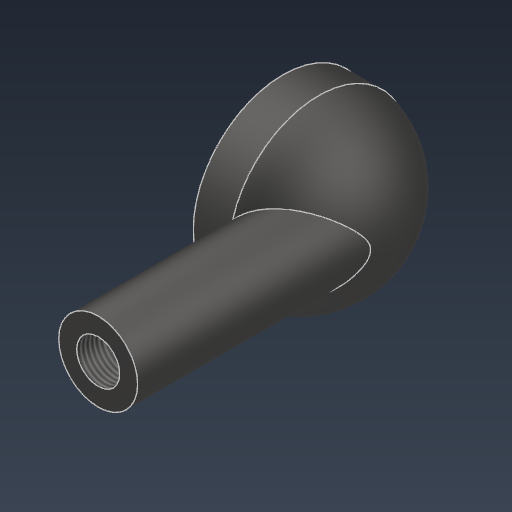
# Autodesk Inventor part: MCEN4000:T4
Saved by Autodesk Inventor 2021 (Build 250183000, 183)
## iProperties
Created: 2020-10-18
Part Number: MCEN4000:T4
Material: STEEL, AISI 1040
Document SubType Name: Modeling
Designer: Eugene Tang
Mass: 302.531 g
Surface Area: 137.328 cm^2
Volume: 38.539 cm^3
Density: 7.85 g/cm^3
Appearance: Semi-Polished
Description: TIE ROD OUTER CUP
Author: Eugene Tang
Autodesk Inventor part; units mm, degrees
ref_plane "YZ Plane" through (0, 0, 0) normal (1, 0, 0) x (0, 1, 0)
ref_plane "XZ Plane" through (0, 0, 0) normal (0, 1, 0) x (-1, 0, 0)
ref_plane "XY Plane" through (0, 0, 0) normal (0, 0, 1) x (1, 0, 0)
sketch "Sketch2" plane through (0, 0, 0) normal (0, 0, 1) x (1, 0, 0)
  circle A0 centre (0, 0) radius 11
  dimension "d1" = 22
  constraints: 1 centre point, 1 coincident
  measures "d1" diameter of A0
extrude "Extrusion1" add sketch "Sketch2" along normal blind 65
sketch "Sketch3" plane through (0, 0, 65) normal (0, 0, 1) x (1, 0, 0)
  circle A0 centre (0, 0) radius 6
  dimension "d4" = 12
  constraints: 1 centre point, 1 coincident
  measures "d4" diameter of A0
extrude "Extrusion2" cut sketch "Sketch3" against normal blind 40
thread "Thread1" size "M12x1.25" class "6H" standard "ISO Metric profile" full length
sketch "Sketch6" plane through (0, 0, 0) normal (0, 1, 0) x (-1, 0, 0)
  line L0 (11, 65) -> (-11, 65) construction
  line L1 (-11.5, -5) -> (56.1068, -5) construction
  line L2 (0, 0) -> (0, -163.2122) construction
  line L3 (8.5, -107.4374) -> (8.5, -5) construction
  line L4 (18.5, -103.8042) -> (18.5, -5) construction
  circle A0 centre (8.5, -5) radius 15
  line L5 (-11.5, -59.4325) -> (-11.5, -5) construction
  circle A1 centre (8.5, -5) radius 20 construction
  line L6 (18.5, -30) -> (18.5, 20) construction
  line L7 (18.5, -30) -> (-11.5, -18.9445) construction
  line L8 (22.2477, -5) -> (22.2477, -11) construction
  line L9 (22.2477, -11) -> (58.2477, -11)
  line L10 (58.2477, -11) -> (58.2477, -5)
  line L11 (23.5, -5) -> (58.2477, -5)
  line L12 (18.5, -30) -> (-11.5, -30) construction
  line L13 (18.5, -25) -> (-11.5, -25) construction
  line L14 (8.5, -20) -> (8.5, -25)
  line L15 (8.5, -25) -> (18.5, -25)
  line L16 (18.5, -25) -> (18.5, -30)
  line L17 (18.5, -30) -> (0, -30)
  arc A2 (-11.5, -5) -> (8.5, -30) centre (14.125, -5) ccw
  line L18 (-11.5, -5) -> (-6.5, -5)
  line L19 (23.5, -5) -> (-6.5, -5)
  point P0 (18.5, -5)
  dimension "d27" = 70
  dimension "d28" = 8.5
  dimension "d30" = 30
  dimension "d31" = 30
  dimension "d32" = 5
  dimension "d33" = 50
  dimension "d34" = 6
  dimension "d35" = 36
  dimension "d36" = 5
  dimension "d37" = 10
  constraints: 36 end point, 10 point on line, 9 point on circle, 5 vertical, 4 tangent, 3 centre point, 3 horizontal, 3 perpendicular, 2 collinear, 2 parallel, 1 coincident, 1 concentric, 1 midpoint, 10 other
  measures "d28" distance between parallel lines of L2 L3
  measures "d30" diameter of A0
  measures "d31" distance between parallel lines of L5 L4
  measures "d32" radial gap between concentric circles of A0 A1
  measures "d33" distance of L6.start L6.end
  measures "d34" distance of L8.start L8.end
  measures "d35" distance between parallel lines of L10 L8
  measures "d36" distance between parallel lines of L13 L12
  measures "d37" distance between parallel lines of L6 L3
revolve "Revolution2" add sketch "Sketch6" angle 360 about axis through (11.5, 0, -5) along (-1, 0, 0) contours A0 L14 L15 L16 L17 A2 L18
sketch "Sketch7" plane through (0, 0, 0) normal (0, 1, 0) x (-1, 0, 0)
  line L0 (23.5, -5) -> (-6.5, -5) projected
  line L1 (18.5, -30) -> (18.5, 20) construction
  line L2 (18.5, -25) -> (-11.5, -25) construction
  line L3 (8.5, -107.4374) -> (8.5, -5) construction
  line L4 (18.5, -5) -> (18.5, -25)
  line L5 (8.5, -25) -> (8.5, -5)
  line L6 (8.5, -5) -> (18.5, -5)
  line L7 (18.5, -25) -> (8.5, -25)
  point P0 (0, 0)
  constraints: 8 end point, 4 collinear, 2 point on line, 1 midpoint
thread "Thread2" size "M40x1.5" class "6H" standard "ISO Metric profile" full length
revolve "Revolution6" cut sketch "Sketch6" angle 360 about axis through (11.5, 0, -5) along (-1, 0, 0) picked at (6.409, -11.3012) contours A0 L19
revolve "Revolution7" cut sketch "Sketch7" angle 360 about axis through (-23.5, 0, -5) along (1, 0, 0)
equation "\"d4\" = Screw_DIA"
equation "\"d5\" = ScrewDEPTH"
equation "\"d16\" = 55deg"
equation "\"Sketch4_Pitch\" = 1.25"
equation "\"d50\" = 55deg"
equation "\"Sketch8_Pitch\" = 1.5"
equation "\"Screw_DIA\" = 12"
equation "\"ScrewDEPTH\" = 40"
body "Solid1"
